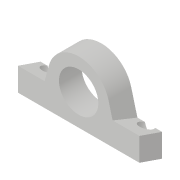
# Autodesk Inventor part: omni wheel shaft holder low channel side attach
Saved by Autodesk Inventor 2018 (Build 220112000, 112)
## iProperties
Created: 2019-02-06
Part Number: omni wheel shaft holder low channel side attach
Material: Generic
Document SubType Name: Modeling
Designer: ball
Density: 1 g/cm^3
Appearance: Default
Author: ball
Autodesk Inventor part; units mm, degrees
ref_plane "YZ Plane" through (0, 0, 0) normal (1, 0, 0) x (0, 1, 0)
ref_plane "XZ Plane" through (0, 0, 0) normal (0, 1, 0) x (-1, 0, 0)
sketch "Sketch1" plane through (0, 0, 0) normal (0, 0, 1) x (1, 0, 0)
  circle A0 centre (0, 0) radius 6.477
  arc A1 (9.8184, 2.6122) -> (-9.8184, 2.6122) centre (0, 0) ccw
  line L0 (0, -10.16) -> (-20, -10.16)
  line L1 (-20, -10.16) -> (-20, -5.08)
  line L2 (0, -5.08) -> (0, -10.16)
  line L3 (0, -10.16) -> (20, -10.16)
  line L4 (20, -10.16) -> (20, -5.08)
  line L5 (0, -5.08) -> (0, -10.16)
  line L6 (-16, -5.08) -> (-16, -10.16) construction
  line L7 (-19.5, -5.08) -> (-19.5, -10.16) construction
  line L8 (-12.5, -5.08) -> (-12.5, -10.16) construction
  line L9 (-11.865, -5.08) -> (-11.865, -10.16) construction
  line L10 (-11.865, -5.08) -> (-9.8184, 2.6122)
  line L11 (16, -5.08) -> (16, -10.16) construction
  line L12 (12.5, -5.08) -> (12.5, -10.16) construction
  line L13 (11.865, -5.08) -> (11.865, -10.16) construction
  line L14 (11.865, -5.08) -> (9.8184, 2.6122)
  line L15 (20, -5.08) -> (11.865, -5.08)
  line L16 (-20, -5.08) -> (-11.865, -5.08)
  dimension "d0" = 12.954
  dimension "d1" = 20.32
  dimension "d3" = 5.08
  dimension "d5" = 5.08
  dimension "d6" = 16
  dimension "d7" = 3.5
  dimension "d8" = 3.5
  dimension "d9" = 0.635
  dimension "d10" = 16
  dimension "d11" = 3.5
  dimension "d12" = 0.635
  constraints: 34 end point, 12 point on line, 9 perpendicular, 4 parallel, 2 centre point, 2 coincident, 2 horizontal, 2 point on circle, 2 tangent
  measures "d0" diameter of A0
  measures "d1" diameter of A1
  measures "d3" distance of L0.end L1.end
  measures "d5" distance of L4.end L3.end
  measures "d6" distance from line of point (0, 0) L6
  measures "d7" distance between parallel lines of L6 L7
  measures "d8" distance between parallel lines of L8 L6
  measures "d9" distance between parallel lines of L9 L8
  measures "d10" distance from line of L11 point (0, 0)
  measures "d11" distance between parallel lines of L11 L12
  measures "d12" distance between parallel lines of L12 L13
ref_plane "Work Plane1" through (-6.9215, -6.9215, 7.4676) normal (0, 0, -1) x (0, 1, 0)
extrude "Extrusion1" add sketch "Sketch1" along normal up to surface (7.4676 mm away)
sketch "Sketch3" plane through (20, -10.16, 0) normal (1, 0, 0) x (0, 0, -1)
  line L0 (-7.4676, 5.08) -> (-7.4676, 0) projected
  line L1 (-7.4676, 0) -> (0, -2.5713)
  line L2 (-7.4676, 0) -> (0.6469, 0) construction
  line L3 (0, 0) -> (0, -2.5713)
  line L4 (0, 0) -> (-7.4676, 0) projected
  line L5 (0, 0) -> (-7.4676, 0)
  point P0 (0, 10.16)
  dimension "d28" = 19
  constraints: 8 end point, 1 collinear, 1 horizontal, 1 point on line, 1 vertical
  measures "d28" angle of L1 L2
extrude "Extrusion2" add sketch "Sketch3" against normal up to surface (40 mm away)
sketch "Sketch4" plane through (20, -5.08, 7.4676) normal (1, 0, 0) x (0, 0, -1)
  line L0 (7.4676, 0) -> (0, 0) projected
  line L1 (7.4676, 0) -> (0, 0)
  line L2 (7.4676, 0) -> (0, 2.5713)
  line L3 (0, 0) -> (0, 7.6922) projected
  line L4 (7.4676, 0) -> (15.3655, 0) construction
  line L5 (0, 7.6922) -> (0, 0) projected
  line L6 (0, 2.5713) -> (0, 0)
  point P0 (7.4676, 5.08)
  dimension "d31" = 161
  constraints: 8 end point, 1 collinear, 1 equal length, 1 horizontal, 1 point on line, 1 vertical
  measures "d31" angle of L4 L2
extrude "Extrusion3" add sketch "Sketch4" against normal blind 10.16
sketch "Sketch5" plane through (-20, -5.08, 0) normal (-1, 0, 0) x (0, 0, 1)
  line L0 (7.4676, 7.6922) -> (7.4676, 0) projected
  line L1 (0, 0) -> (7.4676, 0)
  line L2 (0, 0) -> (7.4676, 2.5713)
  line L3 (0, 0) -> (7.8979, 0) construction
  line L4 (7.4676, 0) -> (7.4676, -5.08) projected
  line L5 (7.4676, 2.5713) -> (7.4676, 0)
  point P0 (0, 5.08)
  dimension "d34" = 19
  constraints: 8 end point, 2 horizontal, 1 equal length, 1 perpendicular, 1 point on line
  measures "d34" angle of L3 L2
extrude "Extrusion4" add sketch "Sketch5" against normal blind 10.16
sketch "Sketch6" plane through (-20, -12.7313, 0) normal (0, -0.9455, 0.3256) x (1, 0, 0)
  line L0 (40, 2.491) -> (40, 10.3889) construction
  line L1 (40, 3.8979) -> (0, 3.8979) construction
  line L2 (0, 7.8979) -> (40, 7.8979) construction
  line L3 (36, 7.8979) -> (36, 0) construction
  line L4 (40, 0) -> (0, 0) construction
  line L5 (40, 7.8979) -> (40, 0) construction
  line L6 (4, 7.8979) -> (4, 0) construction
  line L7 (0, 7.8979) -> (0, 0) construction
  circle A0 centre (36, 3.8979) radius 2.1844
  circle A1 centre (4, 3.8979) radius 2.1844
  point P0 (20, 4.1449)
  dimension "d37" = 4
  dimension "d38" = 4
  dimension "d39" = 4
  dimension "d40" = 4.3688
  dimension "d41" = 4.3688
  constraints: 9 point on line, 6 end point, 2 centre point, 1 perpendicular, 1 vertical
  measures "d37" distance between parallel lines of L1 L2
  measures "d38" distance between parallel lines of L3 L5
  measures "d39" distance between parallel lines of L7 L6
  measures "d40" diameter of A0
  measures "d41" diameter of A1
hole "Hole2" at (16, -11.4623, 3.6855) at (-16, -11.4623, 3.6855) direction (0, 0.9455, -0.3256) diameter 4.3688 end through all
body "Solid1"
